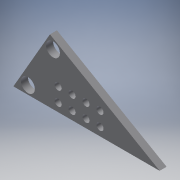
# Autodesk Inventor part: amr4_7
Saved by Autodesk Inventor 2016 (Build 200138000, 138)
## iProperties
Created: 2017-09-19
Part Number: amr4_7
Material: Generic
Document SubType Name: Modeling
Designer: student
Density: 1 g/cm^3
Appearance: Default
Author: student
Autodesk Inventor part; units mm, degrees
ref_plane "YZ Plane" through (0, 0, 0) normal (1, 0, 0) x (0, 1, 0)
ref_plane "XZ Plane" through (0, 0, 0) normal (0, 1, 0) x (-1, 0, 0)
ref_plane "XY Plane" through (0, 0, 0) normal (0, 0, 1) x (1, 0, 0)
sketch "Sketch1" plane through (0, 0, 0) normal (0, 0, 1) x (1, 0, 0)
  circle A0 centre (0, 0) radius 3.175
  circle A1 centre (11.43, -19.7973) radius 3.175
  line L0 (-5.4993, -3.175) -> (5.9307, -22.9723)
  arc A2 (0, 6.35) -> (-5.4993, -3.175) centre (0, 0) ccw
  arc A3 (5.9307, -22.9723) -> (15.0912, -24.9856) centre (11.43, -19.7973) ccw
  line L1 (39.4851, 6.35) -> (0, 6.35)
  arc A4 (0, 6.35) -> (-5.4993, -3.175) centre (0, 0) ccw
  arc A5 (43.1463, -5.1883) -> (39.4851, 6.35) centre (39.4851, 0) ccw
  line L2 (15.0912, -24.9856) -> (43.1463, -5.1883)
  arc A6 (5.9307, -22.9723) -> (15.0912, -24.9856) centre (11.43, -19.7973) ccw
  arc A7 (43.1463, -5.1883) -> (39.4851, 6.35) centre (39.4851, 0) ccw
  circle A8 centre (39.4851, 0) radius 3.175
  line L3 (11.43, -19.7973) -> (39.4851, 0) construction
  circle A9 centre (19.7426, -13.9315) radius 1.5875
  circle A10 centre (26.1654, -9.3992) radius 1.5875
  circle A11 centre (32.1327, -5.1883) radius 1.5875
  dimension "d29" = 6.35
  dimension "d30" = 6.35
  dimension "d36" = 6.35
  dimension "d37" = 3.175
  dimension "d38" = 3.175
  dimension "d39" = 3.175
  constraints: 12 centre point, 12 point on circle, 8 end point, 5 tangent, 3 point on line, 1 coincident, 1 concentric
  measures "d29" diameter of A0
  measures "d30" diameter of A1
  measures "d36" diameter of A8
  measures "d37" diameter of A9
  measures "d38" diameter of A10
  measures "d39" diameter of A11
extrude "Extrusion1" add sketch "Sketch1" along normal blind 3.175
body "Solid1"
